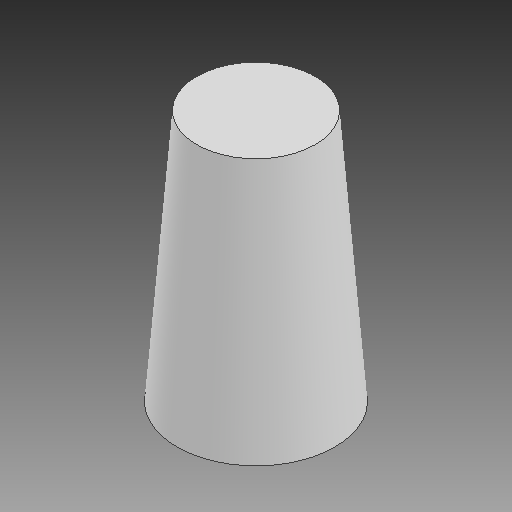
# Autodesk Inventor part: boue
Saved by Autodesk Inventor 2020 (Build 240168000, 168)
## iProperties
Created: 2019-12-27
Part Number: boue
Material: Générique
Document SubType Name: Modeling
Designer: bapti
Density: 1 g/cm^3
Appearance: Par défaut
Mass: 35.4761 g
Surface Area: 490.875 cm^2
Volume: 35.4761 cm^3
Author: bapti
Autodesk Inventor part; units mm, degrees
ref_plane "YZ Plane" through (0, 0, 0) normal (1, 0, 0) x (0, 1, 0)
ref_plane "XZ Plane" through (0, 0, 0) normal (0, 1, 0) x (-1, 0, 0)
ref_plane "XY Plane" through (0, 0, 0) normal (0, 0, 1) x (1, 0, 0)
sketch "Esquisse2" plane through (0, 0, 0) normal (0, 0, 1) x (1, 0, 0)
  line L0 (0, 0) -> (36, 0)
  line L1 (36, 0) -> (27, 115)
  line L2 (27, 115) -> (0, 115)
  line L3 (0, 115) -> (0, 0)
  line L4 (0, 114) -> (25.5737, 114)
  line L5 (25.5737, 114) -> (34.4954, 0)
  dimension "d3" = 27
  dimension "d4" = 36
  dimension "d5" = 115
  dimension "d8" = 1.5
  dimension "d9" = 1
  constraints: 12 end point, 2 horizontal, 2 parallel, 2 point on line, 1 perpendicular
  measures "d3" distance of L1.end L2.end
  measures "d4" distance of L0.start L0.end
  measures "d5" distance of L2.end L0.start
  measures "d8" distance between parallel lines of L1 L5
  measures "d9" distance between parallel lines of L2 L4
revolve "Révolution2" add sketch "Esquisse2" angle 360 about axis through (0, 115, 0) along (0, -1, 0) contours L5 L4 L3 L2 L1 L0
